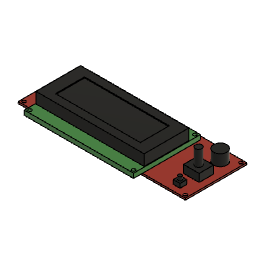
lcd_cover_assembly (Autodesk Fusion 360 archive; units mm, degrees)
design "lcd"
Autodesk Fusion 360 part; units mm, degrees
sketch "Sketch1" plane through (0, 0, 0) normal (0, 0, 1) x (1, 0, 0)
  line L0 (150, 55) -> (150, 0)
  line L1 (150, 0) -> (0, 0)
  line L2 (0, 55) -> (150, 55)
  line L3 (68.5, 32.5) -> (66.3, 32.5) construction
  line L4 (66.3, 32.5) -> (66.3, 23.5)
  line L5 (0, 0) -> (0, 55)
  line L6 (89, 32.5) -> (89, 23.5)
  line L7 (45.8, 32.5) -> (66.3, 32.5)
  line L8 (89, 23.5) -> (68.5, 23.5)
  line L9 (66.3, 23.5) -> (45.8, 23.5)
  line L10 (68.5, 32.5) -> (89, 32.5)
  line L11 (68.5, 23.5) -> (68.5, 32.5)
  line L12 (45.8, 23.5) -> (45.8, 32.5)
  circle A0 centre (2.6, 2.6) radius 1.5
  circle A1 centre (2.6, 52.4) radius 1.5
  circle A2 centre (147.4, 52.4) radius 1.5
  circle A3 centre (147.4, 2.6) radius 1.5
  line L13 (2.6, 52.4) -> (147.4, 52.4) construction
  line L14 (147.4, 52.4) -> (147.4, 2.6) construction
  line L15 (147.4, 2.6) -> (2.6, 2.6) construction
  line L16 (2.6, 2.6) -> (2.6, 52.4) construction
  line L17 (13.5, 52) -> (111.5, 52)
  line L18 (111.5, 52) -> (111.5, -8)
  line L19 (111.5, -8) -> (13.5, -8)
  line L20 (13.5, -8) -> (13.5, 52)
  line L21 (13.5, 42) -> (111.5, 42)
  line L22 (13.5, 2) -> (111.5, 2)
  line L23 (75, 52.4) -> (75, 55) construction
  line L24 (14, 42) -> (14, 2)
  line L25 (111, 42) -> (111, 2)
  circle A4 centre (137, 44.2) radius 6
  line L26 (137, 44.2) -> (137, 8.2) construction
  line L27 (130, 31.3) -> (144, 31.3)
  line L28 (144, 31.3) -> (144, 18.3)
  line L29 (144, 18.3) -> (130, 18.3)
  line L30 (130, 18.3) -> (130, 31.3)
  line L31 (130, 24.8) -> (144, 24.8) construction
  line L32 (134, 11.2) -> (140, 11.2)
  line L33 (140, 11.2) -> (140, 5.2)
  line L34 (140, 5.2) -> (134, 5.2)
  line L35 (134, 5.2) -> (134, 11.2)
  line L36 (140, 8.2) -> (134, 8.2) construction
  circle A5 centre (137, 24.8) radius 3
  line L37 (0, 27.5) -> (150, 27.5) construction
  circle A6 centre (137, 8.2) radius 1.6
  line L38 (0, 8.5) -> (26.5, 8.5)
  line L39 (26.5, 8.5) -> (26.5, 35)
  line L40 (26.5, 35) -> (0, 35)
  line L41 (1, 8.5) -> (1, 35)
  circle A7 centre (16, -5.5) radius 1.5
  circle A8 centre (16, 49.5) radius 1.5
  circle A9 centre (109, -5.5) radius 1.5
  circle A10 centre (109, 49.5) radius 1.5
  line L42 (16, 49.5) -> (16, -5.5) construction
  line L43 (109, 49.5) -> (109, -5.5) construction
  line L44 (109, 49.5) -> (16, 49.5) construction
  line L45 (16, -5.5) -> (109, -5.5) construction
  point P0 (2.6, 27.5)
  dimension "d64" = 9
  dimension "d65" = 9
  dimension "d66" = 20.5
  dimension "d67" = 20.5
  dimension "d70" = 61
  dimension "d71" = 55
  dimension "d72" = 150
  dimension "d77" = 3
  dimension "d78" = 3
  dimension "d79" = 3
  dimension "d80" = 3
  dimension "d83" = 144.8
  dimension "d84" = 49.8
  dimension "d87" = 60
  dimension "d88" = 98
  dimension "d90" = 13.5
  dimension "d91" = 40
  dimension "d94" = 10
  dimension "d108" = 13
  dimension "d111" = 13
  dimension "d112" = 14
  dimension "d113" = 12
  dimension "d114" = 6
  dimension "d115" = 6
  dimension "d116" = 6
  dimension "d1" = 10.6
  dimension "d2" = 2.7
  dimension "d4" = 22.5
  dimension "d5" = 43.2
  dimension "d6" = 19.3
  dimension "d7" = 3.2
  dimension "d12" = 16.7
  dimension "d13" = 26.5
  dimension "d14" = 26.5
  dimension "d19" = 1
  dimension "d20" = 7.5
  dimension "d27" = 3
  dimension "d28" = 3
  dimension "d29" = 3
  dimension "d30" = 3
  dimension "d31" = 93
  dimension "d32" = 2.5
  dimension "d33" = 55
  dimension "d34" = 2.5
  dimension "d36" = 0.5
  dimension "d37" = 0.5
  constraint horizontal L2
  constraint vertical L0
  constraint horizontal L1
  constraint vertical L5
  constraint horizontal L8
  constraint vertical L11
  constraint horizontal L10
  constraint vertical L6
  constraint horizontal L9
  constraint vertical L12
  constraint horizontal L7
  constraint vertical L4
  constraint perpendicular L3 L11
  constraint coincident L1.end L5.start
  constraint horizontal L13
  constraint vertical L14
  constraint horizontal L15
  constraint vertical L16
  constraint coincident A1.centre L13.start
  constraint coincident A0.centre L15.end
  constraint coincident A3.centre L14.end
  constraint coincident A2.centre L13.end
  constraint horizontal L17
  constraint vertical L18
  constraint horizontal L19
  constraint vertical L20
  constraint coincident L20 L21.start
  constraint coincident L18 L21.end
  constraint perpendicular L18 L21
  constraint coincident L20 L22.start
  constraint coincident L18 L22.end
  constraint perpendicular L20 L22
  constraint midpoint L13 L23.start
  constraint midpoint L2 L23.end
  constraint perpendicular L2 L23
  constraint coincident L21 L24.start
  constraint coincident L22 L24.end
  constraint perpendicular L22 L24
  constraint coincident L21 L25.start
  constraint coincident L22 L25.end
  constraint perpendicular L22 L25
  constraint coincident A4.centre L26.start
  constraint vertical L26
  constraint horizontal L27
  constraint vertical L28
  constraint horizontal L29
  constraint vertical L30
  constraint midpoint L30 L31.start
  constraint midpoint L28 L31.end
  constraint symmetric L26 L28 L30
  constraint horizontal L32
  constraint vertical L33
  constraint horizontal L34
  constraint vertical L35
  constraint midpoint L33 L36.start
  constraint midpoint L35 L36.end
  constraint midpoint L26.end L36
  constraint midpoint L31 A5.centre
  constraint midpoint L5 L37.start
  constraint midpoint L0 L37.end
  constraint coincident L16 P0
  constraint midpoint L16 P0
  constraint coincident L37 P0
  constraint coincident L26.end A6.centre
  constraint coincident L5 L38.start
  constraint perpendicular L16 L38
  constraint perpendicular L38 L39
  constraint coincident L5 L40.end
  constraint perpendicular L5 L40
  constraint coincident L38 L41.start
  constraint coincident L40 L41.end
  constraint perpendicular L40 L41
  constraint coincident A8.centre L42.start
  constraint coincident A7.centre L42.end
  constraint vertical L42
  constraint coincident A10.centre L43.start
  constraint coincident A9.centre L43.end
  constraint vertical L43
  constraint horizontal L44
  constraint horizontal L45
  measures "d64" vertical distance of L6.start L6.end
  measures "d65" vertical distance of L7.start L9.end
  measures "d66" horizontal distance of L6.end L8.end
  measures "d67" horizontal distance of L4.end L9.end
  measures "d70" horizontal distance of L6.start L0.start
  measures "d71" distance of L2.start L1.end
  measures "d72" distance of L0.start L2.start
  measures "d77" diameter of A1
  measures "d78" diameter of A2
  measures "d79" diameter of A3
  measures "d80" diameter of A0
  measures "d83" distance of A1.centre A2.centre
  measures "d84" distance of A0.centre A1.centre
  measures "d87" distance of L17.start L19.end
  measures "d88" distance of L17.start L17.end
  measures "d90" horizontal distance of L2.start L17.start
  measures "d91" distance of L21.end L22.end
  measures "d94" distance of L17.end L21.end
  measures "d108" horizontal distance of L0.end L26.end
  measures "d111" distance of L27.end L28.end
  measures "d112" distance of L27.start L27.end
  measures "d113" diameter of A4
  measures "d114" distance of L32.end L33.end
  measures "d115" distance of L32.start L32.end
  measures "d116" diameter of A5
  measures "d1" vertical distance of A0.centre L19.end
  measures "d2" vertical distance of L31.end L37.end
  measures "d4" distance of L2 L10
  measures "d5" distance of L6 L12
  measures "d6" vertical distance of L36.start L37.end
  measures "d7" diameter of A6
  measures "d12" vertical distance of A4.centre L37.end
  measures "d13" distance of L38 L40
  measures "d14" distance of L38.start L38.end
  measures "d19" distance of L5 L41
  measures "d20" distance of L37.start L40
  measures "d27" diameter of A7
  measures "d28" diameter of A9
  measures "d29" diameter of A10
  measures "d30" diameter of A8
  measures "d31" horizontal distance of A7.centre A9.centre
  measures "d32" distance of L18 A9.centre
  measures "d33" vertical distance of A7.centre A8.centre
  measures "d34" distance of L19 A7.centre
  measures "d36" distance of L20 L24
  measures "d37" distance of L18 L25
extrude "Extrude1" add sketch "Sketch1" along normal blind 1.6 contours L0 L1 L2 L5 L17 L18 L20 L40 | L1 L18 L20 L22 | L5 L38 L40 L41 | L1 L5 L20 L38 | L18 L21 L22 L25 | L20 L38 L40 L41 | L20 L22 L24 L38 | L17 L18 L20 L21 | L21 L22 L24 L25 L38 L39 L40 | L20 L24 L38 L40 | L20 L21 L24 L40 | L24 L38 L39 L40 | L4 L7 L9 L12 | L6 L8 L10 L11 | A4 | L27 L28 L29 L30 | L32 L33 L34 L35 | A5 | A6 | A8 | A10
extrude "Extrude2" add sketch "Sketch1" against normal blind 9 contours L4 L7 L9 L12 | L6 L8 L10 L11
extrude "Extrude3" add sketch "Sketch1" along normal blind 4.1 from surface at 1.6 contours L1 L18 L19 L20 | L1 L18 L20 L22 | L18 L21 L22 L25 | L20 L22 L24 L38 | L17 L18 L20 L21 | L21 L22 L24 L25 L38 L39 L40 | L20 L24 L38 L40 | L20 L21 L24 L40 | L24 L38 L39 L40 | L4 L7 L9 L12 | L6 L8 L10 L11
extrude "Extrude4" add sketch "Sketch1" along normal blind 9.8 from surface at 5.7 contours L21 L22 L24 L25 L38 L39 L40 | L24 L38 L39 L40 | L4 L7 L9 L12 | L6 L8 L10 L11
extrude "Extrude5" add sketch "Sketch1" along normal blind 10 from surface at 1.6 contours A4
extrude "Extrude6" add sketch "Sketch1" along normal blind 7 from surface at 1.6 contours L27 L28 L29 L30 | A5
extrude "Extrude7" add sketch "Sketch1" along normal blind 14 from surface at 8.6 contours A5
extrude "Extrude8" add sketch "Sketch1" along normal blind 3.8 from surface at 1.6 contours L32 L33 L34 L35 | A6
extrude "Extrude9" add sketch "Sketch1" along normal blind 7 from surface at 1.6 contours A6
extrude "Extrude10" add sketch "Sketch1" against normal blind 3 contours L20 L38 L40 L41 | L20 L24 L38 L40 | L24 L38 L39 L40
sketch "Sketch2" plane through (0, 0, 15.5) normal (0, 0, 1) x (-1, 0, 0)
  line L0 (-111, -42) -> (-14, -42)
  line L1 (-14, -42) -> (-14, -2)
  line L2 (-14, -2) -> (-111, -2)
  line L3 (-111, -2) -> (-111, -42)
  line L4 (-24.5, -35) -> (-100.5, -35)
  line L5 (-100.5, -35) -> (-100.5, -9)
  line L6 (-100.5, -9) -> (-24.5, -9)
  line L7 (-24.5, -9) -> (-24.5, -35)
  line L8 (-62.5, -42) -> (-62.5, -2) construction
  line L9 (-111, -22) -> (-14, -22) construction
  dimension "d23" = 76
  dimension "d24" = 26
  constraint horizontal L4
  constraint vertical L5
  constraint horizontal L6
  constraint vertical L7
  constraint midpoint L0 L8.start
  constraint midpoint L2 L8.end
  constraint midpoint L3 L9.start
  constraint midpoint L1 L9.end
  constraint symmetric L4 L6 L9
  measures "d23" distance of L5 L7
  measures "d24" distance of L4 L6
extrude "Extrude11" cut sketch "Sketch2" against normal blind 0.8 contours L4 L5 L6 L7
equation "d64 = d65"
equation "d78 = d77"
equation "d79 = d77"
equation "d80 = d77"
equation "d94 = ( d87 - d91 ) / 2"
equation "d28 = d27"
equation "d29 = d27"
equation "d30 = d27"
equation "d32 = ( d88 - d31 ) / 2"
equation "d34 = ( d87 - d33 ) / 2"
equation "d37 = d36"

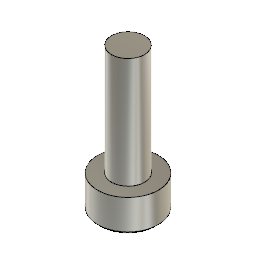
design "base_m3_screw_iso4762"
Autodesk Fusion 360 part; units mm, degrees
sketch "Sketch1" plane through (0, 0, 0) normal (0, 0, 1) x (1, 0, 0)
  circle A0 centre (0, 0) radius 2.75
  circle A1 centre (0, 0) radius 1.5
  circle A2 centre (0, 0) radius 1.25
  line L0 (0.7217, -1.25) -> (1.4434, 0)
  line L1 (1.4434, 0) -> (0.7217, 1.25)
  line L2 (0.7217, 1.25) -> (-0.7217, 1.25)
  line L3 (-0.7217, 1.25) -> (-1.4434, 0)
  line L4 (-1.4434, 0) -> (-0.7217, -1.25)
  line L5 (-0.7217, -1.25) -> (0.7217, -1.25)
  dimension "d1" = 5.5
  dimension "d2" = 3
  dimension "d3" = 2.5
  measures "d1" diameter of A0
  measures "d2" diameter of A1
  measures "d3" diameter of A2
extrude "Extrude1" add sketch "Sketch1" against normal blind 3 contours A0 | A1
extrude "Extrude2" add sketch "Sketch1" along normal blind 10 contours A1 | A2 | A2 L0 L1 | A2 L1 L2 | A2 L0 L5 | A2 L2 L3 | A2 L4 L5 | A2 L3 L4
extrude "Extrude3" add sketch "Sketch1" against normal up to surface (1.5 mm away) contours A2 | A2 L0 L1 | A2 L1 L2 | A2 L0 L5 | A2 L2 L3 | A2 L4 L5 | A2 L3 L4
chamfer "Chamfer1" distance 0.3 angle 45 1 edges at (-2.5639, 0.9944, -3)
equation "d1 = head_dia"
equation "d2 = thread_dia"
equation "d3 = polygon_internal_dia"
equation "d4 = -head_thickness"
equation "d6 = length"
equation "d8 = -polygon_depth"
equation "thread_dia = 3 mm"
equation "length = 10 mm"
equation "head_dia = 5.5 mm"
equation "head_thickness = 3 mm"
equation "polygon_internal_dia = 2.5 mm"
equation "polygon_depth = 1.5 mm"

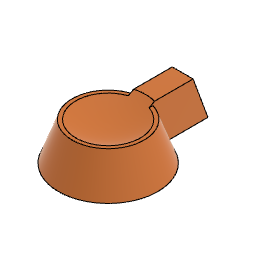
design "lcd_knob"
Autodesk Fusion 360 part; units mm, degrees
sketch "Sketch3" plane through (0, 0, 0) normal (1, 0, 0) x (0, 1, 0)
  line L0 (0, 0) -> (18, 0)
  line L1 (10, 0) -> (7.0154, 8.2)
  line L2 (0, 20) -> (0, 0)
  line L3 (0, 8.2) -> (15.0154, 8.2)
  arc A0 (0, 6) -> (7.5339, 8.2) centre (0, 20) ccw
  line L4 (18, 0) -> (15.0154, 8.2)
  dimension "d22" = 20
  dimension "d23" = 14
  dimension "d24" = 10
  dimension "d31" = 8
  dimension "d1" = 70
  dimension "d9" = 8.2
  constraint coincident L0.start L2.end
  constraint horizontal L0
  constraint perpendicular L0 L2
  constraint parallel L0 L3
  constraint coincident L2.start A0.centre
  constraint coincident L1.start L0
  constraint parallel L1 L4
  constraint coincident L3 L1.end
  constraint coincident A0.end L3
  constraint coincident L2 A0.start
  constraint coincident L2 L3.start
  measures "d22" distance of L0.start L2.start
  measures "d23" radius of A0
  measures "d24" distance of L0.start L1.start
  measures "d31" distance of L1.start L0.end
  measures "d1" angle of L0 L1
  measures "d9" distance of L0 L3
revolve "Revolve1" add sketch "Sketch3" angle 360 about axis through (0, 0, 20) along (0, 0, -1) contours L0 L1 L2 A0 | L1 L2 L3 A0
extrude "Extrude1" add sketch "Sketch3" along normal mid plane 4.2
revolve "Revolve2" cut sketch "Sketch3" angle 360 about axis through (0, 0, 20) along (0, 0, -1) contours L1 L2 L3 A0 | L1 L3 A0
sketch "Sketch4" plane through (0, 0, 8.2) normal (0, 0, 1) x (-1, 0, 0)
  line L0 (-2.1, -7.2353) -> (-2.1, -15.0154)
  line L1 (-2.1, -15.0154) -> (2.1, -15.0154)
  line L2 (2.1, -15.0154) -> (2.1, -7.2353)
  line L3 (2.1, -7.2353) -> (2.1, -5.2353)
  line L4 (2.1, -5.2353) -> (-2.1, -5.2353)
  line L5 (-2.1, -7.2353) -> (-2.1, -5.2353)
  circle A0 centre (0, 0) radius 9.0154
  line L6 (2.1, -7.2353) -> (2.1, -15.0154)
  line L7 (-2.1, -15.0154) -> (-2.1, -7.2353)
  dimension "d13" = 2
  constraint coincident L2.end L3.start
  constraint parallel L2 L3
  constraint perpendicular L3 L4
  constraint parallel L0 L5
  constraint coincident L0.start L5.start
  measures "d13" distance of L2.end L3.end
extrude "Extrude3" cut sketch "Sketch4" against normal blind 0.6 contours L0 L2 L3 L4 L5 A0 L6 L7 picked at (-0.2128, -0.4926)
sketch "Sketch1" plane through (0, 0, 0) normal (0, 0, -1) x (1, 0, 0)
  circle A0 centre (0, 0) radius 3
  circle A1 centre (0, 0) radius 5
  circle A2 centre (0, 0) radius 5.5
  line L0 (4.9749, -0.5) -> (2.958, -0.5)
  line L1 (4.9749, 0.5) -> (2.958, 0.5)
  line L2 (5, 0) -> (0, 0) construction
  line L3 (-2.1, -9.777) -> (-2.1, -18)
  line L4 (-2.1, -18) -> (2.1, -18)
  line L5 (2.1, -18) -> (2.1, -9.777)
  arc A3 (2.1, -9.777) -> (-2.1, -9.777) centre (0, 0) ccw
  dimension "d4" = 6
  dimension "d6" = 0.5
  dimension "d7" = 1
  dimension "d14" = 2
  constraint coincident A0.centre A1.centre
  constraint coincident A1 L0.start
  constraint coincident A0 L0.end
  constraint horizontal L0
  constraint coincident A1 L1.start
  constraint coincident A0 L1.end
  constraint parallel L0 L1
  constraint coincident A1 L2.start
  constraint horizontal L2
  constraint symmetric L0 L1 L2
  constraint concentric A2 A3
  measures "d4" diameter of A0
  measures "d6" distance of A1 A2
  measures "d7" distance of L0.start L1.start
  measures "d14" distance of A0 A1
extrude "Extrude2" cut sketch "Sketch1" against normal blind 4.6 contours A0 | A0 A1 L0 L1 | A2 picked at (3.6642, -0.1114)
chamfer "Chamfer1" distance 0.4 distance2 0.5 1 edges at (-3, 0, 0) measured on face at (-4.3242, 0, 0)
chamfer "Chamfer2" distance 0.225 distance2 0.9 2 edges at (-5, 0, 0) (-5.1278, -1.9889, 0) measured on face at (-4.4575, 0, 0) measured on face at (0.7, 12.518, 0)

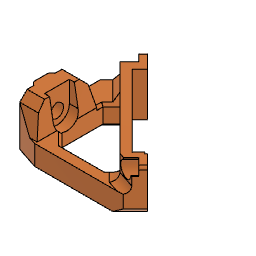
design "lcd_support_a"
Autodesk Fusion 360 part; units mm, degrees
sketch "base" plane through (0, 0, 0) normal (0, 0, 1) x (1, 0, 0)
  line L0 (6.3887, 41.8887) -> (46.4817, 1.7958)
  line L1 (0, 35.5) -> (0, 0)
  line L2 (44.6859, 0) -> (49.593, 4.907)
  line L3 (0, 0) -> (44.6859, 0)
  line L4 (43.3277, 0) -> (3.9139, 39.4139)
  line L5 (9.5, 45) -> (0, 35.5)
  line L6 (9, 0) -> (9, 25)
  line L7 (9, 25) -> (0, 25)
  line L8 (0, 17.45) -> (-1.4, 16.05)
  line L9 (-1.4, 16.05) -> (-1.4, 9.95)
  line L10 (-1.4, 9.95) -> (0, 8.55)
  line L11 (-1.4, 13) -> (0, 13) construction
  line L12 (-0.225, 8.775) -> (0, 8.775)
  line L13 (-0.225, 17.225) -> (0, 17.225)
  line L14 (0, 3) -> (9, 0)
  line L15 (11.9395, 42.5605) -> (0, 30.621) construction
  line L16 (47.1534, 7.3466) -> (39.8069, 0) construction
  line L17 (26.4352, 21.8423) -> (4.593, 0) construction
  line L18 (12.3638, 35.9137) -> (15.4751, 39.0249)
  line L19 (15.4751, 39.0249) -> (9.5, 45)
  line L20 (41.2137, 7.0637) -> (44.325, 10.175)
  line L21 (44.325, 10.175) -> (49.593, 4.907)
  line L22 (41.2137, 7.0637) -> (12.3638, 35.9137)
  dimension "d2480" = 0
  dimension "d2481" = 0
  dimension "d2482" = 0
  dimension "d2483" = 0
  dimension "d2497" = 0
  dimension "d2498" = 0
  dimension "d2499" = 0
  dimension "d2500" = 0
  dimension "d32_1" = 8.9
  dimension "d33_1" = 1.4
  dimension "d35_1" = 45
  dimension "d91" = 9
  dimension "d117" = 0.225
  dimension "d118" = 0.225
  dimension "d241" = 12
  dimension "d255" = 10
  dimension "d288" = 45
  dimension "d338" = 56.7
  dimension "d341" = 4
  dimension "d342" = 49.8
  dimension "d344" = 5
  dimension "d345" = 4.4
  dimension "d372" = 45
  dimension "d373" = 9.5
  dimension "d417" = 32
  dimension "d418" = 3.5
  constraint coincident L1.end L3.start
  constraint horizontal L3
  constraint perpendicular L1 L3
  constraint perpendicular L6 L7
  constraint coincident L1 L8.start
  constraint parallel L1 L9
  constraint coincident L1 L10.end
  constraint midpoint L9 L11.start
  constraint coincident L1 L11.end
  constraint perpendicular L9 L11
  constraint perpendicular L8 L10
  constraint coincident L3 L6.start
  constraint perpendicular L3 L6
  constraint coincident L10 L12.start
  constraint coincident L1 L12.end
  constraint perpendicular L1 L12
  constraint coincident L8 L13.start
  constraint coincident L1 L13.end
  constraint perpendicular L1 L13
  constraint coincident L1.start L5.end
  constraint coincident L7.end L1
  constraint coincident L1 L14.start
  constraint coincident L1 L15.end
  constraint coincident L3 L16.end
  constraint coincident L3 L17.end
  constraint perpendicular L18 L19
  constraint coincident L5.start L19.end
  constraint perpendicular L20 L21
  constraint coincident L2.end L21.end
  constraint collinear L19 L21
  constraint coincident L16.start L21
  constraint coincident L15.start L19
  constraint perpendicular L15 L19
  constraint perpendicular L16 L21
  constraint coincident L0.end L2
  constraint coincident L0.start L5
  constraint coincident L4.end L5
  constraint perpendicular L4 L5
  constraint perpendicular L2 L21
  constraint perpendicular L20 L22
  constraint perpendicular L5 L19
  constraint coincident L4.start L3
  constraint midpoint L0 L17.start
  constraint coincident L0 L18.start
  measures "d32_1" vertical distance of L8.start L10.end
  measures "d33_1" distance of L1 L9
  measures "d35_1" angle of L1 L10
  measures "d91" distance of L1.end L6
  measures "d117" vertical distance of L8.start L13.end
  measures "d118" vertical distance of L10.end L12.end
  measures "d241" vertical distance of L7.end L11.start
  measures "d255" vertical distance of L11.start L14.start
  measures "d288" angle of L1 L5
  measures "d338" distance of L5.start L2.end
  measures "d341" distance of L16.start L20.end
  measures "d342" distance of L15.start L16.start
  measures "d344" distance of L15.start L18.end
  measures "d345" distance of L18.start L18.end
  measures "d372" vertical distance of L1.end L5.start
  measures "d373" horizontal distance of L1.start L5.start
  measures "d417" vertical distance of L5.start L11.start
  measures "d418" distance of L4 L22
extrude "Extrude15" add sketch "base" against normal blind 8 contours L0 L5 L18 L19 | L0 L2 L3 L4 L5 L22 | L1 L3 L4 L5 L6 L7 | L0 L2 L20 L21 | L1 L6 L7 L14
extrude "Extrude16" add sketch "base" along normal blind 11.4 contours L1 L6 L7 L14 | L1 L8 L9 L10 L12 L13
extrude "Extrude17" add sketch "base" along normal blind 9.6 contours L0 L2 L3 L4 L5 L22
sketch "Sketch16" plane through (27.25, 27.25, 0) normal (0.707107, 0.707107, 0) x (-0.707107, 0.707107, 0)
  line L0 (-28.1477, 9.6) -> (-28.1477, 0) construction
  line L1 (-24.1477, 9.6) -> (-24.1477, 0)
  circle A0 centre (-28.1477, 6.3) radius 1.6
  line L2 (16.6523, 9.6) -> (16.6523, 0)
  line L3 (21.6523, 0) -> (21.6523, 9.6) construction
  line L4 (-28.1477, 6.3) -> (21.6523, 6.3) construction
  circle A1 centre (21.6523, 6.3) radius 1.6
  circle A2 centre (-28.1477, 6.3) radius 2.9
  circle A3 centre (21.6523, 6.3) radius 2.9
  line L5 (-24.9477, 9.6) -> (-24.9477, -8)
  line L6 (-26.8965, 9.15) -> (-26.0971, 8.3506)
  line L7 (20.4011, 9.15) -> (19.6017, 8.3506)
  line L8 (-26.8965, 9.15) -> (-26.8965, 9.6)
  line L9 (20.4011, 9.15) -> (20.4011, 9.6)
  line L10 (-24.1477, 0) -> (-31.5977, 0)
  line L11 (-31.5977, 0) -> (-31.5977, -8)
  line L12 (-31.5977, -8) -> (-24.1477, -8)
  line L13 (-24.1477, -8) -> (-24.1477, 0)
  line L14 (16.6523, 0) -> (25.1023, 0)
  line L15 (25.1023, 9.6) -> (-30.6373, 9.6)
  line L16 (-31.0477, 6.3) -> (-31.5977, 6.3)
  line L17 (-31.0477, 6.3) -> (-28.1477, 6.3) construction
  line L18 (21.6523, 6.3) -> (24.5523, 6.3) construction
  line L19 (24.5523, 6.3) -> (25.1023, 6.3)
  line L20 (16.6523, 0) -> (16.6523, -8)
  line L21 (22.4523, 7.6856) -> (21.6523, 8.1475)
  line L22 (21.6523, 8.1475) -> (20.8523, 7.6856)
  line L23 (-28.9477, 7.6856) -> (-28.1477, 8.1475)
  line L24 (-28.1477, 8.1475) -> (-27.3477, 7.6856)
  line L25 (-30.6373, 9.6) -> (-31.5977, 9.6)
  line L26 (25.1023, 0) -> (16.6523, 0)
  line L27 (-31.5977, 0) -> (-31.5977, 9.6)
  line L28 (25.1023, 0) -> (25.1023, 9.6)
  line L29 (-24.1477, 0) -> (-31.5977, 0)
  point P0 (16.6523, 0)
  point P1 (25.1023, 0)
  point P2 (-28.1477, 0)
  point P3 (-28.1477, 0)
  point P4 (21.6523, 0)
  point P5 (21.6523, 0)
  dimension "d297" = 3.2
  dimension "d298" = 6.3
  dimension "d301" = 3.2
  dimension "d305" = 5.8
  dimension "d306" = 5.8
  dimension "d328" = 0.45
  dimension "d331" = 0.45
  dimension "d348" = 3.2
  dimension "d374" = 45
  dimension "d378" = 45
  dimension "d393" = 60
  dimension "d394" = 60
  constraint coincident L0 A0.centre
  constraint coincident A0.centre L4.start
  constraint coincident L3 L4.end
  constraint perpendicular L3 L4
  constraint coincident L4.end A1.centre
  constraint concentric A0 A2
  constraint concentric A1 A3
  constraint coincident A2 L6.end
  constraint coincident A3 L7.end
  constraint tangent A3 L7
  constraint tangent A2 L6
  constraint coincident P0 L2.end
  constraint coincident L5.end L12
  constraint coincident L1.end L10.start
  constraint horizontal L4
  constraint coincident L2.start L15
  constraint coincident L3.end L15
  constraint coincident L9.end L15
  constraint perpendicular L9 L15
  constraint coincident L5.start L15
  constraint coincident L1.start L15
  constraint coincident L0.start L15
  constraint coincident L8.end L15
  constraint parallel L1 L13
  constraint perpendicular L5 L15
  constraint perpendicular L8 L15
  constraint perpendicular L0 L15
  constraint coincident A2 L16.start
  constraint coincident L16.end L27
  constraint perpendicular L16 L27
  constraint parallel L16 L17
  constraint coincident A3 L18.end
  constraint coincident L19.end L28
  constraint perpendicular L19 L28
  constraint parallel L18 L19
  constraint parallel L2 L20
  constraint coincident A1 L21.start
  constraint tangent A1 L21
  constraint coincident A1 L22.end
  constraint tangent A1 L22
  constraint coincident L3 L21.end
  constraint coincident L21.end L22.start
  constraint coincident A0 L23.start
  constraint coincident L0 L23.end
  constraint coincident A0 L24.end
  constraint tangent A0 L24
  constraint tangent A0 L23
  constraint coincident P3 L0.end
  constraint coincident P5 P4
  measures "d297" diameter of A0
  measures "d298" vertical distance of A0.centre L10.end
  measures "d301" diameter of A1
  measures "d305" diameter of A2
  measures "d306" diameter of A3
  measures "d328" distance of L6.start L8.end
  measures "d331" distance of L7.start L9.end
  measures "d348" distance of L0.start L5.start
  measures "d374" angle of L7 L15
  measures "d378" angle of L6 L15
  measures "d393" angle of L3 L22
  measures "d394" angle of L0 L23
extrude "Extrude27" add sketch "Sketch16" against normal up to surface (4.4 mm away) contours L1 L5 L10 L15 L29 | A2 L5 L6 L8 L10 L15 L16 L27 L29 | A2 L6 L8 L15 L16 L25 L27 | A2 | L2 A3 L7 L9 L14 L15 L19 L26 L28 | A3 L7 L9 L15 L19 L28 | A3
extrude "Extrude28" cut sketch "Sketch16" against normal blind 0.8 contours L1 L5 L10 L15 L29 | L5 L10 L12 L13 L29
extrude "Extrude29" add sketch "Sketch16" against normal blind 7.4784 contours L2 A3 L7 L9 L14 L15 L19 L26 L28 | A3 L7 L9 L15 L19 L28 | A3
extrude "Extrude30" cut sketch "Sketch16" against normal blind 20 from surface at -2.5 contours A2 L6 L8 L15 L16 L25 L27 | A2 | A0 | A0 L23 L24 | A3 L7 L9 L15 L19 L28 | A3 | A1 | A1 L21 L22
fillet "Fillet1" radius 1 2 edges at (48.7091, 4.0232, 9.6) (8.6161, 44.1161, 9.6)
sketch "Sketch20" plane through (27.25, 27.25, 0) normal (0.707107, 0.707107, 0) x (-0.707107, 0.707107, 0)
  arc A0 (-30.5977, 9.6) -> (-31.5977, 8.6) centre (-30.5977, 8.6) ccw
  line L0 (-31.5977, 8.6) -> (-31.5977, -8)
  line L1 (-31.5977, -8) -> (-24.9477, -8)
  line L2 (-24.9477, -8) -> (-24.9477, 9.6)
  line L3 (-24.9477, 9.6) -> (-30.5977, 9.6)
  arc A1 (-28.9477, 7.6856) -> (-27.3477, 7.6856) centre (-28.1477, 6.3) ccw
  line L4 (-28.9477, 7.6856) -> (-28.1477, 8.1475)
  line L5 (-28.1477, 8.1475) -> (-27.3477, 7.6856)
  line L6 (-24.1477, 9.6) -> (-24.1477, -8)
  line L7 (-24.9477, -8) -> (-24.9477, 9.6)
  line L8 (-24.9477, -8) -> (-31.5977, -8)
  line L9 (-24.1477, -8) -> (-24.9477, -8)
  arc A2 (-28.9477, 7.6856) -> (-27.3477, 7.6856) centre (-28.1477, 6.3) ccw
  line L10 (-24.1477, 0.8) -> (-26.3477, 0.8)
  line L11 (-26.3477, 0.8) -> (-26.3477, -8)
  dimension "d405" = 1.8
  dimension "d406" = 5.5
  constraint coincident L6 L10.start
  constraint coincident L8 L11.end
  constraint perpendicular L1 L11
  constraint perpendicular L6 L10
  measures "d405" horizontal distance of A1.centre L11.end
  measures "d406" vertical distance of A1.centre L10.end
extrude "Extrude36" cut sketch "Sketch20" against normal blind 1.5 contours L2 L6 L7 L9 L10 | L1 L2 L7 L8 L10 L11
draft "Draft2" angle 45 neutral plane through (26.1893, 26.1893, 0) pull (0.707107, 0.707107, 0) 1 faces at (45.0085, 8.4072, 0.8)
sketch "frame_hole" plane through (9, 0, 0) normal (1, 0, 0) x (0, 1, 0)
  line L0 (0, 0) -> (25, 0)
  line L1 (25, 0) -> (25, 11.4)
  line L2 (25, 11.4) -> (0, 11.4)
  circle A0 centre (13, 2.9) radius 2.65
  line L3 (0, 0) -> (25, 0)
  circle A1 centre (13, 2.9) radius 5
  line L4 (11.675, 5.195) -> (12.6363, 5.75)
  line L5 (12.6363, 5.75) -> (13.3637, 5.75)
  line L6 (13.3637, 5.75) -> (14.325, 5.195)
  line L7 (0, 11.4) -> (25, 11.4)
  line L8 (18, 2.9) -> (18, 11.4)
  line L9 (8, 2.9) -> (8, 11.4)
  line L10 (16.05, 11.4) -> (9.95, 11.4)
  line L11 (13, 2.9) -> (13, 11.4) construction
  line L12 (0, 11.4) -> (0, 0)
  point P0 (13, 5.75)
  dimension "d183" = 10
  dimension "d184" = 5.3
  dimension "d186" = 0.2
  dimension "d246" = 150
  dimension "d280" = 8.5
  constraint concentric A0 A1
  constraint coincident A0 L4.start
  constraint coincident A0 L6.end
  constraint coincident A1 L8.start
  constraint coincident L2 L8.end
  constraint coincident A1 L9.start
  constraint coincident L2 L9.end
  constraint tangent A1 L8
  constraint tangent A1 L9
  constraint coincident A0.centre A1.centre
  constraint coincident L10 L11.end
  constraint midpoint L10 L11.end
  constraint perpendicular L7 L11
  constraint perpendicular L2 L9
  constraint perpendicular L7 L8
  constraint tangent A0 L4
  constraint tangent A0 L6
  constraint perpendicular L5 L11
  constraint midpoint L5 P0
  constraint coincident L11 P0
  measures "d183" diameter of A1
  measures "d184" diameter of A0
  measures "d186" distance of A0 L5
  measures "d246" angle of L4 L5
  measures "d280" distance of A0.centre L7
extrude "Extrude19" cut sketch "frame_hole" against normal blind 28 contours A0 | A0 L4 L5 L6
extrude "Extrude20" cut sketch "frame_hole" along normal blind 9 from surface at -4 contours L0 L3 A1 | L0 L3 A1 | L2 A1 L7 L8 L9 L10 | A0 | A0 L4 L5 L6
chamfer "Chamfer16" distance 2 distance2 11.4 2 edges at (9, 21.5, 11.4) (9, 4, 11.4) measured on face at (4.6667, 22.6667, 11.4) measured on face at (4.6667, 22.6667, 11.4)
sketch "poly_holes" plane through (0, 0, 0) normal (0, 0, 1) x (-1, 0, 0)
  line L0 (-43.3277, 0) -> (-3.9139, -39.4139)
  line L1 (-9, 0) -> (-43.3277, 0)
  line L2 (0, -35.5) -> (0, -25)
  line L3 (-15, -5) -> (-32.7153, -5)
  line L4 (-9, -27.5294) -> (-12.3991, -30.9286)
  line L5 (-9, -25) -> (-9, -27.5294)
  line L6 (-9, -11) -> (-15, -5)
  line L7 (-9, -11) -> (-9, -17.0731)
  line L8 (-3.9139, -39.4139) -> (0, -35.5)
  line L9 (-9, -25) -> (-9, -17.0731)
  line L10 (-9, 0) -> (-43.3277, 0)
  line L11 (-32.7153, -5) -> (-35.5215, -7.8062)
  line L12 (-47.8252, -3.1393) -> (-44.6859, 0)
  dimension "d273" = 6
  dimension "d381" = 5
  dimension "d384" = 45
  dimension "d396" = 12
  dimension "d397" = 12
  constraint horizontal L3
  constraint parallel L5 L7
  constraint coincident L5.start L9.start
  constraint coincident L7.end L9.end
  constraint parallel L5 L9
  constraint coincident L0 L11.end
  constraint coincident L0 L4.end
  constraint perpendicular L0 L4
  constraint perpendicular L0 L11
  measures "d273" distance of L3 L6.start
  measures "d381" distance of L3 L10
  measures "d384" angle of L3 L6
  measures "d396" distance of L4 L8
  measures "d397" distance of L11 L12
extrude "Extrude21" cut sketch "poly_holes" against normal blind 15
chamfer "Chamfer21" distance 1 angle 45 10 edges at (10.6996, 29.229, -8) (23.8577, 5, -8) (23.8577, 5, 0) (10.6996, 29.229, 0) (13.0365, 6.9635, 0) (12, 8, -8) (9, 19.2647, -8) (34.1184, 6.4031, 0) (34.1184, 6.4031, -8) (9, 26.2647, 0)
sketch "frame_hole_chamfer" plane through (0, 0, 0) normal (-1, 0, 0) x (0, -1, 0)
  line L0 (-35.5, -8) -> (-3, -8)
  line L1 (-3, 11.4) -> (-8.775, 11.4)
  line L2 (-8.775, 11.4) -> (-8.775, 0)
  line L3 (-8.775, 0) -> (-17.225, 0)
  line L4 (-17.225, 0) -> (-17.225, 11.4)
  line L5 (-17.225, 11.4) -> (-25, 11.4)
  line L6 (-25, 11.4) -> (-25, 0)
  line L7 (-25, 0) -> (-25, 11.4)
  line L8 (-23, 8.4) -> (-20, 11.4)
  line L9 (-6, 11.4) -> (-3, 8.4)
  line L10 (-3, 8.4) -> (-23, 8.4) construction
  line L11 (-3, 8.4) -> (-1, 0)
  arc A0 (-14.325, 5.195) -> (-11.675, 5.195) centre (-13, 2.9) ccw
  line L12 (-8, 11.4) -> (-18, 11.4)
  line L13 (-13, 2.9) -> (-13, 11.4) construction
  line L14 (-23, 8.4) -> (-25, 0)
  line L15 (-25, 0) -> (-35.5, 0)
  line L16 (-35.5, 0) -> (-35.5, -8)
  line L17 (-8, 11.4) -> (-0.6667, 11.4)
  line L18 (-8.9269, 0) -> (0, 0)
  line L19 (-25, 0) -> (-17.0731, 0)
  line L20 (-0.6667, 11.4) -> (0, 0)
  dimension "d263" = 10
  dimension "d281" = 45
  dimension "d282" = 2
  dimension "d283" = 3
  constraint horizontal L10
  constraint coincident A0.centre L13.start
  constraint midpoint L12 L13.end
  constraint coincident L5 L8.end
  constraint coincident L1 L9.start
  constraint symmetric L8 L9 L13
  constraint coincident L11.end L18
  constraint coincident L6.end L19
  constraint coincident L6.end L7.start
  constraint symmetric L11 L13 L14
  measures "d263" horizontal distance of L9.end L13.end
  measures "d281" angle of L5 L8
  measures "d282" distance of L8.end L12.end
  measures "d283" distance of L8.end L10
extrude "Extrude22" cut sketch "frame_hole_chamfer" against normal blind 12.5 contours L1 L9 L11 L17 L18 L20 | L5 L6 L7 L8 L14
chamfer "Chamfer20" distance 3 angle 45 2 edges at (4.75, 40.25, -8) (47.1394, 2.4535, -8)
extrude "Extrude26" add 1 faces at (-0.4667, 11.9833, 0) along direction (0, 0, -1) blind 5
draft "Draft3" angle 45 neutral plane through (0, 35.5, 0) pull (-1, 0, 0) 1 faces at (-0.4667, 11.9833, -5)
sketch "Sketch19" plane through (0, 0, 9.6) normal (0, 0, 1) x (-1, 0, 0)
  line L0 (-10.2071, -44.2929) -> (-8.4393, -42.5251)
  line L1 (-8.4393, -42.5251) -> (-11.0565, -39.908)
  line L2 (-11.0565, -39.908) -> (-7.2381, -36.0896)
  line L3 (-7.2381, -36.0896) -> (-40.6825, -2.6452)
  line L4 (-40.6825, -2.6452) -> (-44.5009, -6.4635)
  line L5 (-48.8858, -5.6142) -> (-44.8907, -9.6093)
  line L6 (-44.8907, -9.6093) -> (-44.325, -9.0436)
  line L7 (-44.325, -9.0436) -> (-43.7593, -9.6093)
  line L8 (-43.7593, -9.6093) -> (-41.2137, -7.0637)
  line L9 (-12.3638, -35.9137) -> (-15.4751, -39.0249)
  line L10 (-5, -10.35) -> (-5, -15.65)
  line L11 (-5, -15.65) -> (-46.3917, -1.7058)
  line L12 (-47.4363, -3.5282) -> (-43.9081, 0)
  line L13 (-47.8252, -3.1393) -> (-44.6859, 0)
  line L14 (-15.4751, -39.0249) -> (-10.2071, -44.2929)
  line L15 (-44.6859, 0) -> (-40.4433, 0)
  line L16 (-41.2137, -7.0637) -> (-12.3638, -35.9137)
  line L17 (-43.3277, 0) -> (-36.2286, -7.0991)
  line L18 (-48.8858, -5.6142) -> (-49.593, -4.907)
  line L19 (-44.8907, -9.6093) -> (-48.8858, -5.6142)
  point P0 (-45.8099, -1.9018)
  dimension "d421" = 4.8
  constraint coincident L10.end L11.start
  constraint coincident L11.end L13
  constraint coincident L12 P0
  constraint coincident L11 P0
  measures "d421" distance of L5 P0
extrude "Extrude35" cut sketch "Sketch19" against normal up to surface (9.6 mm away)
fillet "Fillet2" radius 3 2 edges at (42.7952, 2.9175, 0) (37.7136, 5.6141, 0)
chamfer "Chamfer25" distance 2 angle 45 1 edges at (7.8029, 35.5248, 0)
chamfer "Chamfer24" distance 2.89 angle 45 1 edges at (4.1083, 39.2194, 6.3)
ref_plane "WorkPlane1" through (2.5, 13, 4.65) normal (1, 0, 0) x (0, 0, -1)
sketch "selective_infill" plane through (2.5, 0, 0) normal (1, 0, 0) x (0, 1, 0)
  line L0 (8.159, 5.55) -> (8.26, 5.55)
  line L1 (8.26, 5.55) -> (8.26, 0.25)
  line L2 (8.26, 0.25) -> (8.159, 0.25)
  line L3 (8.159, 0.25) -> (8.159, 5.55)
  line L4 (17.841, 5.55) -> (17.74, 5.55)
  line L5 (17.74, 5.55) -> (17.74, 0.25)
  line L6 (17.74, 0.25) -> (17.841, 0.25)
  line L7 (17.841, 0.25) -> (17.841, 5.55)
  line L8 (8.26, 2.9) -> (17.74, 2.9) construction
  arc A0 (11.675, 5.195) -> (14.325, 5.195) centre (13, 2.9) ccw
  arc A1 (11.675, 5.195) -> (14.325, 5.195) centre (13, 2.9) ccw
  dimension "d247" = 0.101
  dimension "d248" = 0.101
  dimension "d249" = 2.09
  constraint horizontal L0
  constraint vertical L1
  constraint horizontal L2
  constraint vertical L3
  constraint horizontal L4
  constraint vertical L5
  constraint horizontal L6
  constraint vertical L7
  constraint midpoint L1 L8.start
  constraint midpoint L5 L8.end
  constraint horizontal L8
  constraint midpoint L8 A0.centre
  constraint tangent L6 A1
  constraint tangent L2 A0
  measures "d247" distance of L5.end L6.end
  measures "d248" distance of L1.end L2.end
  measures "d249" distance of L5 A0
extrude "Extrude24" cut sketch "selective_infill" along normal mid plane 0.101
move_body "Move1" [suppressed]
mirror "Mirror1" [suppressed]
equation "m5_hole = 5.3 mm"
equation "m5_head = 10 mm"
equation "d52 = ( 0.45 * 2 ) * 1 mm"
equation "layer_height = 0.20 mm"
equation "extrusion_width = 0.45 mm"
equation "num_perimeters = 3"
equation "selective_infill_horizontal_height = layer_height"
equation "perimeters_width = extrusion_width + ( ( num_perimeters - 1 ) * 0.4071 ) * 1 mm"
equation "vslot_profile_width = 8.9 mm"
equation "vslot_profile_height = 1.4 mm"
equation "num_top_bottom = 5"
equation "top_bottom_thickness = num_top_bottom * layer_height"
equation "d32_1 = vslot_profile_width"
equation "d33_1 = vslot_profile_height"
equation "d117 = extrusion_width / 2"
equation "d118 = extrusion_width / 2"
equation "d158 = 4.75 mm"
equation "d159 = d158 / 2"
equation "d183 = m5_head"
equation "d184 = m5_hole"
equation "d186 = layer_height"
equation "d249 = extrusion_width + ( 4 * 0.41 ) * 1 mm"
equation "m3_hole = 3.2 mm"
equation "d297 = m3_hole"
equation "d301 = m3_hole"
equation "m3_head = 5.8 mm"
equation "d305 = m3_head"
equation "d306 = m3_head"
equation "d328 = extrusion_width"
equation "d331 = extrusion_width"
equation "d338 = 55 mm + ( 2 * 1 ) * 1 mm - 0.3 mm"
equation "d397 = d396"
equation "d412 = m3_head / 2 - 0.01 mm"
equation "d218 = -top_bottom_thickness * 2"
equation "d219 = -top_bottom_thickness - layer_height - 0.001 mm"
equation "d221 = perimeters_thickness * 2"
equation "d222 = perimeters_thickness * 2"
equation "d223 = layer_height * 5 + 0.001 mm"
equation "d224 = d223"
equation "d227 = -perimeters_thickness * 2"
equation "d230 = perimeters_thickness * 2"
equation "d231 = perimeters_thickness * 2"
named bodies: "lcd_support_b"
